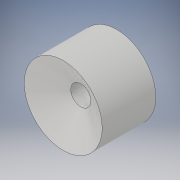
# Autodesk Inventor part: 85mmWheel
Saved by Autodesk Inventor 2018 (Build 220112000, 112)
## iProperties
Created: 2019-06-09
Part Number: 85mmWheel
Material: Generic
Document SubType Name: Modeling
Designer: anirudh
Density: 1 g/cm^3
Appearance: Default
Author: anirudh
Autodesk Inventor part; units mm, degrees
ref_plane "YZ Plane" through (0, 0, 0) normal (1, 0, 0) x (0, 1, 0)
ref_plane "XZ Plane" through (0, 0, 0) normal (0, 1, 0) x (-1, 0, 0)
ref_plane "XY Plane" through (0, 0, 0) normal (0, 0, 1) x (1, 0, 0)
sketch "Sketch2" plane through (0, 0, 0) normal (1, 0, 0) x (0, 1, 0)
  line L0 (85, 29.25) -> (85, -29.25)
  line L1 (53.5, 0) -> (53.5, 10)
  line L2 (53.5, 10) -> (85, 29.25)
  line L3 (53.5, 0) -> (53.5, -10)
  line L4 (53.5, -10) -> (85, -29.25)
  line L5 (42.5, 0) -> (42.5, -56.6203)
  point P0 (0, 0)
  dimension "d6" = 11
  dimension "d7" = 10
  constraints: 12 end point, 2 vertical
  measures "d6" distance of L5.start L1.start
  measures "d7" distance of L1.start L1.end
revolve "Revolution1" add sketch "Sketch2" angle 360 about axis through (0, 42.5, 0) along (0, 0, -1)
body "Solid1"
